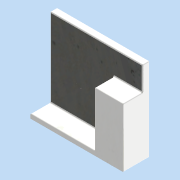
# Autodesk Inventor part: Wand
Saved by Autodesk Inventor 2021 (Build 250183000, 183)
## iProperties
Created: 2024-03-17
Part Number: Wand
Material: Generic
Document SubType Name: Modeling
Designer: Nokia
Density: 1 g/cm^3
Appearance: Snow
Author: Nokia
Autodesk Inventor part; units mm, degrees
ref_plane "YZ Plane" through (0, 0, 0) normal (1, 0, 0) x (0, 1, 0)
ref_plane "XZ Plane" through (0, 0, 0) normal (0, 1, 0) x (-1, 0, 0)
ref_plane "XY Plane" through (0, 0, 0) normal (0, 0, 1) x (1, 0, 0)
sketch "Sketch1" plane through (0, 0, 0) normal (0, 0, 1) x (1, 0, 0)
  line L0 (0, 0) -> (1330, 0)
  line L1 (1330, 0) -> (1330, 1150)
  line L2 (1330, 1150) -> (1950, 1150)
  line L3 (0, 0) -> (0, -100)
  line L4 (0, -100) -> (1950, -100)
  line L5 (1950, -100) -> (1950, 1150)
  dimension "d1" = 1150
  dimension "d2" = 620
  dimension "d3" = 100
  dimension "d18" = 1950
  constraints: 12 end point, 2 perpendicular, 2 vertical, 1 horizontal, 1 parallel
  measures "d1" distance of L0.end L1.end
  measures "d2" distance of L1.end L2.end
  measures "d3" distance of L0.start L3.end
  measures "d18" distance between parallel lines of L5 L3
extrude "Extrusion1" add sketch "Sketch1" against normal blind 565
sketch "Sketch2" plane through (0, 0, 0) normal (0, 1, 0) x (1, 0, 0)
  line L0 (1950, 565) -> (0, 565) projected
  line L1 (0, 565) -> (0, 415)
  line L2 (0, 0) -> (0, 565) projected
  line L3 (0, 415) -> (1950, 415)
  line L4 (1950, 0) -> (1950, 565) projected
  line L5 (1950, 415) -> (1950, 565)
  line L6 (1950, 565) -> (0, 565)
  dimension "d6" = 150
  constraints: 8 end point, 2 perpendicular, 2 point on line
  measures "d6" distance of L0.end L1.end
extrude "Extrusion2" add sketch "Sketch2" along normal blind 1655
fillet "Fillet1" radius 20 23 edges at (975, 1655, -415) (975, 1655, -565) (1950, 777.5, -565) (1950, 1402.5, -415) (1640, 1150, -415) (1950, 1150, -207.5) (1330, 1150, -207.5) (1330, 575, 0) (1330, 575, -415) (1330, 0, -207.5) (665, 0, 0) (665, 0, -415) (975, -100, -565) (0, 827.5, -415) (0, 777.5, -565) (0, 1655, -490) (1950, 1655, -490) (1950, -100, -282.5) (1640, 1150, 0) (1950, 525, 0) (975, -100, 0) (0, 0, -207.5) (0, -100, -282.5)
sketch "Sketch3" plane through (20, 1635, -415) normal (0, 0, 1) x (1, 0, 0)
  circle A0 centre (530, -1018) radius 13.6015
  circle A1 centre (633, -1056) radius 12.3693
  point P0 (-20, -1635)
  constraints: 2 centre point
hole "Hole1" at (550, 617, -415) at (653, 579, -415) direction (0, 0, -1) diameter 10.106 depth 39 tip angle 118 thread size "M12x1.75" class "6H" standard "ISO Metric profile"
sketch "Sketch4" plane through (0, 0, 0) normal (0, 0, 1) x (1, 0, 0)
  point P0 (0, 0)
body "Solid1"
